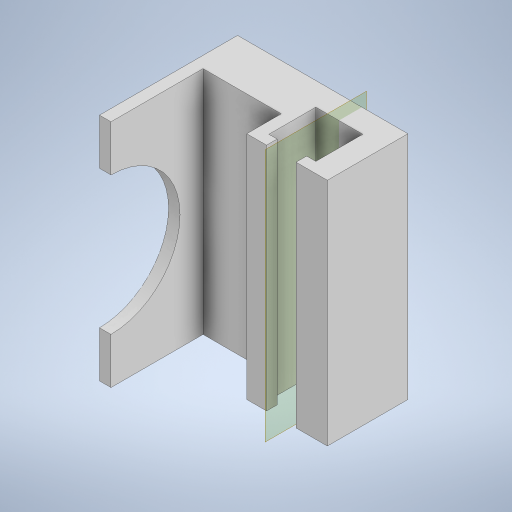
# Autodesk Inventor part: Schiene
Saved by Autodesk Inventor 2024 (Build 280153000, 153)
## iProperties
Created: 2024-01-24
Part Number: Schiene
Material: Generisch
Document SubType Name: Modeling
Designer: mariu
Density: 1 g/cm^3
Appearance: Vorgabe
Author: mariu
Autodesk Inventor part; units mm, degrees
ref_plane "YZ Plane" through (0, 0, 0) normal (1, 0, 0) x (0, 1, 0)
ref_plane "XZ Plane" through (0, 0, 0) normal (0, 1, 0) x (-1, 0, 0)
ref_plane "XY Plane" through (0, 0, 0) normal (0, 0, 1) x (1, 0, 0)
sketch "Skizze1" plane through (0, 0, 0) normal (0, 0, 1) x (1, 0, 0)
  line L0 (0, 0) -> (22, 0)
  line L1 (22, 0) -> (22, 10)
  line L2 (22, 10) -> (0, 10)
  line L3 (0, 10) -> (0, 0)
  dimension "d0" = 22
  dimension "d1" = 10
  constraints: 8 end point, 2 parallel, 1 horizontal, 1 perpendicular
  measures "d0" distance of L2.end L1.end
  measures "d1" distance of L1.end L0.end
extrude "Extrusion1" add sketch "Skizze1" along normal blind 50
sketch "Skizze3" plane through (22, 0, 0) normal (1, 0, 0) x (0, 0, -1)
  line L0 (-50, 0) -> (-50, 10) projected
  line L1 (0, 0) -> (0, 10) projected
  line L2 (-50, 10) -> (0, 10)
  line L3 (0, 10) -> (0, 5)
  line L4 (0, 5) -> (-50, 5)
  line L5 (-50, 5) -> (-50, 10)
  constraints: 8 end point, 2 parallel, 1 horizontal, 1 midpoint, 1 perpendicular
extrude "Extrusion2" add sketch "Skizze3" along normal blind 15
sketch "Skizze4" plane through (22, 5, 0) normal (0, -1, 0) x (1, 0, 0)
  line L0 (-22, 50) -> (15, 50) projected
  line L1 (15, 50) -> (10.2, 50)
  line L2 (10.2, 50) -> (10.2, 0)
  line L3 (10.2, 0) -> (15, 0)
  line L4 (15, 0) -> (15, 50)
  line L5 (0, 0) -> (0, 50) projected
  point P0 (-22, 0)
  dimension "d6" = 10.2
  constraints: 8 end point, 2 parallel, 1 horizontal, 1 perpendicular
  measures "d6" distance between parallel lines of L5 L2
extrude "Extrusion3" add sketch "Skizze4" along normal blind 5
sketch "Skizze5" plane through (0, 0, 0) normal (0, -1, 0) x (1, 0, 0)
  line L0 (22, 0) -> (22, 50) projected
  line L1 (22, 50) -> (17, 50)
  line L2 (17, 50) -> (17, 0)
  line L3 (17, 0) -> (22, 0)
  line L4 (22, 0) -> (22, 50)
  line L5 (32.2, 50) -> (32.2, 0) projected
  line L6 (37, 0) -> (37, 50) projected
  line L7 (32.2, 50) -> (37, 50)
  line L8 (37, 50) -> (37, 0)
  line L9 (37, 0) -> (32.2, 0)
  line L10 (32.2, 0) -> (32.2, 50)
  point P0 (0, 0)
  dimension "d9" = 5
  constraints: 16 end point, 4 parallel, 2 horizontal, 2 perpendicular
  measures "d9" distance between parallel lines of L0 L2
extrude "Extrusion4" add sketch "Skizze5" along normal blind 10
sketch "Skizze6" plane through (32.2, 5, 0) normal (-1, 0, 0) x (0, 0, 1)
  line L0 (50, 5) -> (50, -15) projected
  line L1 (0, 5) -> (0, -15) projected
  line L2 (50, -15) -> (0, -15)
  line L3 (0, -15) -> (0, -10.2)
  line L4 (0, -10.2) -> (50, -10.2)
  line L5 (50, -10.2) -> (50, -15)
  point P0 (0, -5)
  point P1 (0, -15)
  point P2 (50, -10.2)
  dimension "d12" = 4.8
  constraints: 8 end point, 2 parallel, 1 horizontal, 1 perpendicular, 1 point on line
  measures "d12" distance between parallel lines of L4 L2
extrude "Extrusion5" add sketch "Skizze6" along normal blind 2
ref_plane "Arbeitsebene1" through (27, 0, 0) normal (-1, 0, 0) x (0, 0, 1)
mirror "Spiegeln1" about plane through (27, 0, 0) normal (-1, 0, 0) of "Extrusion5"
sketch "Skizze7" plane through (0, -10, 0) normal (0, -1, 0) x (1, 0, 0)
  line L0 (0, 50) -> (37, 50) projected
  line L1 (17, 0) -> (17, 50) projected
  line L2 (37, 50) -> (17, 50)
  line L3 (17, 50) -> (17, 0)
  line L4 (17, 0) -> (37, 0)
  line L5 (37, 0) -> (37, 50)
  point P0 (0, 0)
  constraints: 8 end point, 2 parallel, 1 horizontal, 1 perpendicular
extrude "Extrusion6" cut sketch "Skizze7" against normal blind 2.5
sketch "Skizze8" plane through (0, 0, 0) normal (-1, 0, 0) x (0, 0, 1)
  point P0 (0, 0)
sketch "Skizze9" plane through (0, 0, 0) normal (-1, 0, 0) x (0, 0, 1)
  line L0 (50, -20) -> (0, -20)
  line L1 (0, -20) -> (0, 30)
  line L2 (0, 30) -> (50, 30)
  line L3 (50, 30) -> (50, -20)
  line L4 (0, 0) -> (50, 0) projected
  line L5 (50, 10) -> (50, 0) projected
  point P0 (50, 5)
  dimension "d17" = 50
  dimension "d18" = 50
  dimension "d19" = 20
  dimension "d20" = 0
  constraints: 8 end point, 2 parallel, 1 horizontal, 1 midpoint, 1 perpendicular
  measures "d17" distance of L1.end L2.end
  measures "d18" distance of L0.end L1.end
  measures "d19" distance between parallel lines of L4 L0
  measures "d20" distance from line of point (50, 5) L3
extrude "Extrusion7" add sketch "Skizze9" against normal blind 2.5
sketch "Skizze10" plane through (0, -20, 0) normal (-1, 0, 0) x (0, 0, 1)
  circle A0 centre (25, 0) radius 15
  line L0 (0, 0) -> (50, 0) projected
  point P0 (0, 20)
  point P1 (25, 0)
  point P2 (10, 0)
  point P3 (40, 0)
  dimension "d23" = 30
  constraints: 1 centre point, 1 coincident, 1 midpoint
  measures "d23" diameter of A0
extrude "Extrusion8" cut sketch "Skizze10" against normal blind 2.5 contours L0 A0 picked at (21.7322, 7.6351)
sketch "Skizze11" plane through (17, 0, 0) normal (-1, 0, 0) x (0, 0, 1)
  line L0 (0, -7.5) -> (50, -7.5) projected
  line L1 (0, 0) -> (0, -7.5) projected
  line L2 (50, -7.5) -> (0, -7.5)
  line L3 (0, -7.5) -> (0, 0)
  line L4 (0, 0) -> (50, 0)
  line L5 (50, 0) -> (50, -7.5)
  constraints: 8 end point, 2 parallel, 1 horizontal, 1 perpendicular
extrude "Extrusion9" cut sketch "Skizze11" against normal blind 2.5
sketch "Skizze12" plane through (2.5, 0, 0) normal (1, 0, 0) x (0, 0, -1)
  line L0 (-50, 10) -> (-50, -7.5) projected
  line L1 (0, 30) -> (0, -20) projected
  line L2 (-50, 10) -> (0, 10)
  line L3 (0, 10) -> (0, 30)
  line L4 (0, 30) -> (-50, 30)
  line L5 (-50, 30) -> (-50, 10)
  point P0 (0, 0)
  point P1 (0, 10)
  constraints: 8 end point, 2 parallel, 1 horizontal, 1 perpendicular
extrude "Extrusion10" cut sketch "Skizze12" against normal blind 10
